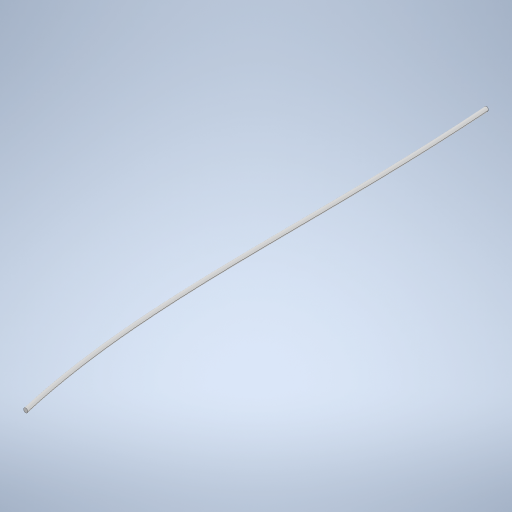
# Autodesk Inventor part: wire
Saved by Autodesk Inventor 2024.2 (Build 282272000, 272)
## iProperties
Created: 2025-02-11
Part Number: wire
Material: Generic
Document SubType Name: Modeling
Designer: Tom
Density: 1 g/cm^3
Appearance: Default
Author: Tom
Autodesk Inventor part; units mm, degrees
ref_plane "YZ Plane" through (0, 0, 0) normal (1, 0, 0) x (0, 1, 0)
ref_plane "XZ Plane" through (0, 0, 0) normal (0, 1, 0) x (-1, 0, 0)
ref_plane "XY Plane" through (0, 0, 0) normal (0, 0, 1) x (1, 0, 0)
sketch "Sketch1" plane through (0, 0, 0) normal (1, 0, 0) x (0, 1, 0)
  line L0 (0, 0) -> (2.5963, -8.7567) construction
  line L1 (2.5963, -8.7567) -> (1.2274, -19.9445) construction
  line L2 (1.2274, -19.9445) -> (2.1715, -32.5956) construction
  spline S0 degree 3 poles (0, 0) (2.5963, -8.7567) (1.2274, -19.9445) (2.1715, -32.5956) knots 1 1 1 1 2 2 2 2
  constraints: 3 other
sketch "Sketch2" plane through (0, 0, 0) normal (0, 0, 1) x (1, 0, 0)
  circle A0 centre (0, 0) radius 0.1524
  dimension "d0" = 0.3048
  constraints: 1 centre point, 1 coincident
  measures "d0" diameter of A0
sweep "Sweep1" add profiles "Sketch2" path "Sketch1"
body "Solid1"
